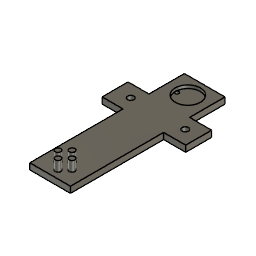
cameraholder (Autodesk Fusion 360 design; units mm, degrees)
part number: 2026-06-05-13-18-55-107
Autodesk Fusion 360 part; units mm, degrees
sketch "スケッチ1" plane through (0, 0, 0) normal (0, 0, 1) x (1, 0, 0)
  line L0 (0, 0) -> (32.4214, 0)
  line L1 (32.4214, 0) -> (32.4214, 74.2625)
  line L2 (32.4214, 74.2625) -> (0, 74.2625)
  line L3 (0, 74.2625) -> (0, 0)
  line L4 (32.4214, 74.2625) -> (50, 74.2625)
  line L5 (50, 74.2625) -> (50, 95)
  line L6 (50, 95) -> (32.4214, 95)
  line L7 (32.4214, 95) -> (32.4214, 74.2625)
  line L8 (0, 74.2625) -> (-16.6488, 74.2625)
  line L9 (-16.6488, 74.2625) -> (-16.6488, 95)
  line L10 (-16.6488, 95) -> (0, 95)
  line L11 (0, 95) -> (0, 74.2625)
  line L12 (0, 95) -> (32.4214, 95)
  line L13 (32.4214, 95) -> (32.4214, 74.2625)
  line L14 (32.4214, 74.2625) -> (0, 74.2625)
  line L15 (0, 74.2625) -> (0, 95)
  circle A0 centre (16.2107, 6.34) radius 2.25
  circle A1 centre (16.2107, 17.54) radius 2.25
  circle A2 centre (16.2107, 17.54) radius 2.25
  circle A3 centre (16.2107, 6.34) radius 2.25
  circle A4 centre (16.2107, 6.34) radius 2.25
  circle A5 centre (16.2107, 17.54) radius 2.25
  circle A6 centre (16.2107, 17.54) radius 2.25
  circle A7 centre (16.2107, 6.34) radius 2.25
  circle A8 centre (21.783, 11.9123) radius 2.25
  circle A9 centre (10.583, 11.9123) radius 2.25
  circle A10 centre (21.783, 11.9123) radius 2.25
  circle A11 centre (21.783, 11.9123) radius 2.25
  circle A12 centre (10.583, 11.9123) radius 2.25
  circle A13 centre (10.583, 11.9123) radius 2.25
  circle A14 centre (10.583, 11.9123) radius 2.25
  circle A15 centre (21.783, 11.9123) radius 2.25
  circle A16 centre (-4.4, 85) radius 1.25
  circle A17 centre (39.5, 85) radius 1.25
  circle A18 centre (-5, 85) radius 1.25
  circle A19 centre (38.9, 85) radius 1.25
  line L16 (39.504, 86.25) -> (38.9019, 86.25)
  line L17 (38.9019, 86.25) -> (38.9019, 83.75)
  line L18 (38.9019, 83.75) -> (39.504, 83.75)
  line L19 (39.504, 83.75) -> (39.504, 86.25)
  line L20 (-5.0028, 86.25) -> (-4.4097, 86.25)
  line L21 (-4.4097, 86.25) -> (-4.4097, 83.75)
  line L22 (-4.4097, 83.75) -> (-5.0028, 83.75)
  line L23 (-5.0028, 83.75) -> (-5.0028, 86.25)
  dimension "d1" = 4.5
  dimension "d2" = 4.5
  dimension "d3" = 11.2
  dimension "d4" = 4.5
  dimension "d5" = 4.5
  dimension "d6" = 11.2
  dimension "d7" = 4.5
  dimension "d8" = 4.5
  dimension "d9" = 11.2
  dimension "d10" = 4.5
  dimension "d11" = 4.5
  dimension "d12" = 11.2
  dimension "d13" = 4.5
  dimension "d14" = 4.5
  dimension "d15" = 11.2
  dimension "d16" = 4.5
  dimension "d17" = 4.5
  dimension "d18" = 11.2
  dimension "d19" = 4.5
  dimension "d20" = 4.5
  dimension "d21" = 11.2
  dimension "d22" = 4.5
  dimension "d23" = 4.5
  dimension "d24" = 11.2
  dimension "d25" = 2.5
  dimension "d26" = 2.5
  dimension "d27" = 43.9
  dimension "d28" = 2.5
  dimension "d29" = 2.5
  constraint horizontal L0
  constraint vertical L1
  constraint horizontal L2
  constraint vertical L3
  constraint coincident L0.start L3.end
  constraint horizontal L4
  constraint vertical L5
  constraint horizontal L6
  constraint vertical L7
  constraint horizontal L8
  constraint vertical L9
  constraint horizontal L10
  constraint vertical L11
  constraint horizontal L12
  constraint vertical L13
  constraint horizontal L14
  constraint vertical L15
  constraint horizontal L16
  constraint vertical L17
  constraint horizontal L18
  constraint vertical L19
  constraint coincident A19 L17.end
  constraint coincident A17 L16.start
  constraint horizontal L20
  constraint vertical L21
  constraint horizontal L22
  constraint vertical L23
  constraint coincident A16 L21.end
  constraint coincident A18 L20.start
  measures "d1" diameter of A0
  measures "d2" diameter of A1
  measures "d3" distance of A0.centre A1.centre
  measures "d4" diameter of A3
  measures "d5" diameter of A2
  measures "d6" distance of A0.centre A1.centre
  measures "d7" diameter of A7
  measures "d8" diameter of A5
  measures "d9" distance of A0.centre A1.centre
  measures "d10" diameter of A4
  measures "d11" diameter of A6
  measures "d12" distance of A0.centre A1.centre
  measures "d13" diameter of A15
  measures "d14" diameter of A12
  measures "d15" distance of A8.centre A9.centre
  measures "d16" diameter of A10
  measures "d17" diameter of A13
  measures "d18" distance of A8.centre A9.centre
  measures "d19" diameter of A11
  measures "d20" diameter of A9
  measures "d21" distance of A8.centre A9.centre
  measures "d22" diameter of A8
  measures "d23" diameter of A14
  measures "d24" distance of A8.centre A9.centre
  measures "d25" diameter of A16
  measures "d26" diameter of A17
  measures "d27" horizontal distance of A16.centre A17.centre
  measures "d28" diameter of A18
  measures "d29" diameter of A19
extrude "押し出し1" add sketch "スケッチ1" along normal blind 5
sketch "スケッチ2" plane through (0, 0, 0) normal (0, 0, -1) x (1, 0, 0)
  circle A0 centre (16.2107, -17.54) radius 2.25
  circle A1 centre (10.583, -11.9123) radius 2.25
  circle A2 centre (16.2107, -6.34) radius 2.25
  arc A3 (-4.9899, -83.75) -> (-5.0028, -86.25) centre (-5, -85) ccw
  line L0 (-4.9899, -83.75) -> (-4.4097, -83.75)
  arc A4 (-4.4097, -86.25) -> (-4.4097, -83.75) centre (-4.4, -85) ccw
  line L1 (-4.4097, -86.25) -> (-4.4097, -86.25)
  line L2 (-4.4097, -86.25) -> (-5.0028, -86.25)
  line L3 (38.9019, -83.75) -> (39.504, -83.75)
  arc A5 (39.504, -86.25) -> (39.504, -83.75) centre (39.5, -85) ccw
  line L4 (39.504, -86.25) -> (38.9019, -86.25)
  arc A6 (38.9019, -83.75) -> (38.9019, -86.25) centre (38.9, -85) ccw
  circle A7 centre (21.783, -11.9123) radius 2.25
  line L5 (0, 0) -> (0, -74.2625)
  line L6 (0, -74.2625) -> (-16.6488, -74.2625)
  line L7 (-16.6488, -74.2625) -> (-16.6488, -95)
  line L8 (-16.6488, -95) -> (50, -95)
  line L9 (50, -95) -> (50, -74.2625)
  line L10 (50, -74.2625) -> (32.4214, -74.2625)
  line L11 (32.4214, -74.2625) -> (32.4214, 0)
  line L12 (32.4214, 0) -> (0, 0)
  circle A8 centre (10.583, -11.9123) radius 2.25
  circle A9 centre (16.2107, -6.34) radius 2.25
  circle A10 centre (21.783, -11.9123) radius 2.25
  circle A11 centre (16.2107, -17.54) radius 2.25
  constraint concentric A1 A8
  constraint concentric A2 A9
  constraint concentric A7 A10
  constraint concentric A0 A11
extrude "押し出し2" add sketch "スケッチ2" against normal blind 13 contours A0 A11 | A1 A8 | A2 A9 | A7 A10
move_face "面をオフセット1" offset -0.05 4 faces at (18.4495, 6.116, 7.6667) (24.0302, 12.0245, 10.3333) (18.4495, 17.316, 7.6667) (12.8302, 12.0245, 10.3333)
sketch "スケッチ3" plane through (0, 0, 5) normal (0, 0, 1) x (-1, 0, 0)
  circle A0 centre (-16.2107, -17.54) radius 2.2
  circle A1 centre (-10.583, -11.9123) radius 2.2
  circle A2 centre (-16.2107, -6.34) radius 2.2
  arc A3 (5.0028, -86.25) -> (4.9899, -83.75) centre (5, -85) ccw
  line L0 (5.0028, -86.25) -> (4.4097, -86.25)
  line L1 (4.4097, -86.25) -> (4.4097, -86.25)
  arc A4 (4.4097, -83.75) -> (4.4097, -86.25) centre (4.4, -85) ccw
  line L2 (4.4097, -83.75) -> (4.9899, -83.75)
  line L3 (-39.504, -83.75) -> (-38.9019, -83.75)
  arc A5 (-38.9019, -86.25) -> (-38.9019, -83.75) centre (-38.9, -85) ccw
  line L4 (-38.9019, -86.25) -> (-39.504, -86.25)
  arc A6 (-39.504, -83.75) -> (-39.504, -86.25) centre (-39.5, -85) ccw
  circle A7 centre (-21.783, -11.9123) radius 2.2
  line L5 (0, -74.2625) -> (0, 0)
  line L6 (0, 0) -> (-32.4214, 0)
  line L7 (-32.4214, 0) -> (-32.4214, -74.2625)
  line L8 (-32.4214, -74.2625) -> (-50, -74.2625)
  line L9 (-50, -74.2625) -> (-50, -95)
  line L10 (-50, -95) -> (16.6488, -95)
  line L11 (16.6488, -95) -> (16.6488, -74.2625)
  line L12 (16.6488, -74.2625) -> (0, -74.2625)
  circle A8 centre (4.5, -85) radius 2.5
  circle A9 centre (-38.9, -85) radius 2.5
  dimension "d35" = 5
  constraint concentric A5 A9
  measures "d35" diameter of A9
extrude "押し出し3" cut sketch "スケッチ3" against normal blind 6 contours A8 | A9
move_face "面をオフセット2" offset 0.05 4 faces at (12.7721, 11.6933, 7.6667) (18.3998, 17.3209, 7.6667) (18.3998, 6.1209, 7.6667) (23.9721, 11.6933, 7.6667)
sketch "スケッチ4" plane through (0, 0, 0) normal (0, 0, -1) x (1, 0, 0)
  circle A0 centre (38.9, -85) radius 2.5
  circle A1 centre (-4.5, -85) radius 2.5
  line L0 (0, 0) -> (0, -74.2625)
  line L1 (0, -74.2625) -> (-16.6488, -74.2625)
  line L2 (-16.6488, -74.2625) -> (-16.6488, -95)
  line L3 (-16.6488, -95) -> (50, -95)
  line L4 (50, -95) -> (50, -74.2625)
  line L5 (50, -74.2625) -> (32.4214, -74.2625)
  line L6 (32.4214, -74.2625) -> (32.4214, 0)
  line L7 (32.4214, 0) -> (0, 0)
  line L8 (0, -95) -> (32.4214, -95)
  line L9 (32.4214, -95) -> (32.4214, -123.2444)
  line L10 (32.4214, -123.2444) -> (0, -123.2444)
  line L11 (0, -123.2444) -> (0, -95)
  constraint horizontal L8
  constraint vertical L9
  constraint horizontal L10
  constraint vertical L11
  constraint coincident L3 L8.start
extrude "押し出し4" add sketch "スケッチ4" against normal blind 5 contours L3 L8 L9 L10 L11
hole "穴1" at (16.3211, 109.6527, 5) direction (0, 0, -1) diameter 20 depth 2.5 tip angle 180
hole "穴2" at (24.8415, 109.7629, 2.5) direction (0, 0, -1) diameter 3 depth 2.5 tip angle 180
hole "穴3" at (7.8139, 109.5886, 2.5) direction (0, 0, -1) diameter 3 depth 2.5 tip angle 180
